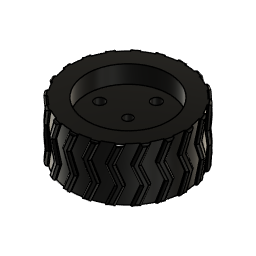
Back Wheel v9 (Autodesk Fusion 360 design; units mm, degrees)
Autodesk Fusion 360 part; units mm, degrees
note: some values were not read from the file. Set by a fixed rule: which sketch regions a step uses.
sketch "Main" plane through (0, 0, 0) normal (0, 0, 1) x (1, 0, 0)
  circle A0 centre (0, 0) radius 16
  dimension "d4" = 32
  constraint coincident A0.centre origin
  measures "d4" diameter of A0
extrude "Extrude2" add sketch "Main" along normal blind 15
sketch "Internal pocket" plane through (0, 0, 15) normal (0, 0, 1) x (-1, 0, 0)
  circle A0 centre (0, 0) radius 16
  circle A1 centre (0, 0) radius 11.6
  dimension "d49" = 23.2
  constraint coincident A0.centre A1.centre
  measures "d49" diameter of A1
sketch "External pocket" plane through (0, 0, 0) normal (0, 0, -1) x (1, 0, 0)
  circle A0 centre (0, 0) radius 11.25
  circle A1 centre (0, 0) radius 16
  dimension "d21" = 22.5
  constraint coincident A0.centre A1.centre
  measures "d21" diameter of A0
extrude "Extrude6" cut sketch "External pocket" against normal blind 5 contours A0
fillet "Fillet2" radius 2 1 edges at (-10.4887, -4.0682, 0)
sketch "Grooves" plane through (0, 0, 0) normal (1, 0, 0) x (0, 1, 0)
  line L0 (16, 0) -> (16, 15)
  line L1 (-16, 0) -> (-16, 15)
  line L2 (-2, 10) -> (0, 5)
  line L3 (0, 5) -> (-2, 0)
  line L4 (0, 10) -> (2, 5)
  line L5 (2, 5) -> (0, 0)
  line L6 (0, 0) -> (-2, 0)
  line L7 (0, 0) -> (-16, 0)
  line L8 (16, 0) -> (0, 0)
  line L9 (0, 15) -> (-16, 15)
  line L10 (16, 15) -> (0, 15)
  line L11 (0, 10) -> (2, 15)
  line L12 (-2, 10) -> (0, 15)
  dimension "d38" = 2
  dimension "d39" = 5
  dimension "d40" = 2
  dimension "d64" = 5
  constraint parallel L2 L4
  constraint parallel L3 L5
  constraint horizontal L2.end L4.end
  constraint coincident L3.end L6.end
  constraint horizontal L6
  constraint coincident L6 L5.end
  constraint horizontal L2.start L4.start
  constraint coincident L10 L11.end
  constraint coincident L10 L9.start
  constraint parallel L11 L12
  constraint vertical L4.end L11.end
  constraint vertical L2.start L3.end
  constraint vertical L5.end L2.end
  measures "d38" horizontal distance of L2.end L3.end
  measures "d39" vertical distance of L2.end L3.end
  measures "d40" distance of L2.end L4.end
  measures "d64" vertical distance of L2.start L2.end
extrude "Extrude9" add sketch "Grooves" along normal blind 0.8 from the near side of the face at (15.9205, -1.5931, 10) contours L2 L3 L4 L5 L6 L7 L10 L11 L12
fillet "Fillet4" radius 0.5 6 edges at (16.7686, -1.002, 2.4951) (16.7686, -1.002, 0) (16.7686, 1.002, 2.5049) (16.7686, 1.002, 7.4951) (16.7686, -1.002, 7.5049) (16.7686, 1.002, 15)
fillet "Fillet4" radius 0.5 2 edges at (16.7686, -1.002, 12.4951) (16.7686, 1.002, 12.5049)
pattern_circular "C-Pattern1" count 20 over 360 about axis through (0, 0, 1.75) along (0, 0, 1) of "Extrude9", "Fillet4"
extrude "Extrude10" cut sketch "Internal pocket" against normal blind 5 contours A1
sketch "Flange Holes" plane through (0, 0, 10) normal (0, 0, 1) x (-1, 0, 0)
  circle A0 centre (0, 0) radius 11.6
  circle A1 centre (8, 0) radius 1.4
  circle A2 centre (0, 8) radius 1.4
  circle A3 centre (-8, 0) radius 1.4
  circle A4 centre (0, -8) radius 1.4
  circle A5 centre (0, 0) radius 1.25
  dimension "d52" = 2.8
  dimension "d53" = 8
  dimension "d55" = 360
  dimension "d57" = 2.5
  constraint horizontal A0.centre A1.centre
  constraint concentric A0 A5
  measures "d52" diameter of A1
  measures "d53" distance of A0.centre A1.centre
  measures "d57" diameter of A5
extrude "Extrude11" cut sketch "Flange Holes" against normal through all contours A1 | A2 | A3 | A4
extrude "Extrude12" cut sketch "Flange Holes" against normal blind 2 contours A5
